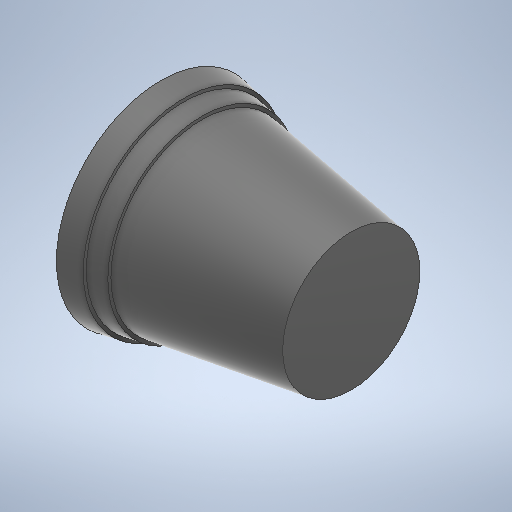
# Autodesk Inventor part: Tanque
Saved by Autodesk Inventor 2025.3 (Build 293356000, 356)
## iProperties
Created: 2025-11-02
Part Number: Tanque
Material: Plástico ABS
Document SubType Name: Modeling
Designer: PAVILION
Density: 1.06 g/cm^3
Appearance: Suave - Blanco
Author: PAVILION
Autodesk Inventor part; units mm, degrees
ref_plane "YZ Plane" through (0, 0, 0) normal (1, 0, 0) x (0, 1, 0)
ref_plane "XZ Plane" through (0, 0, 0) normal (0, 1, 0) x (-1, 0, 0)
ref_plane "XY Plane" through (0, 0, 0) normal (0, 0, 1) x (1, 0, 0)
sketch "Boceto1" plane through (0, 0, 0) normal (0, 1, 0) x (-1, 0, 0)
  line L0 (0, 450) -> (0, -450)
  line L1 (1250, 685) -> (1250, -685)
  line L2 (1250, 685) -> (1100, 658.551)
  line L3 (1100, 658.551) -> (1100, 638.551)
  line L4 (1100, 638.551) -> (980, 617.3917)
  line L5 (980, 617.3917) -> (980, 597.3917)
  line L6 (980, 597.3917) -> (0, 450)
  line L7 (1250, 668.5436) -> (1114.356, 644.6259)
  line L8 (1114.356, 644.6259) -> (1114.356, 624.6259)
  line L9 (1114.356, 624.6259) -> (994.356, 603.4667)
  line L10 (994.356, 603.4667) -> (994.356, 583.4667)
  line L11 (994.356, 583.4667) -> (20, 435)
  line L12 (20, 435) -> (20, 0)
  line L13 (0, 0) -> (20, 0)
  line L14 (1250, 685) -> (1250, 668.5436)
  line L15 (0, 0) -> (1250, 0)
  dimension "d0" = 900
  dimension "d1" = 1370
  dimension "d2" = 1250
  dimension "d3" = 100
  dimension "d4" = 100
  dimension "d5" = 150
  dimension "d6" = 20
  dimension "d7" = 120
  dimension "d8" = 20
  dimension "d9" = 20
  dimension "d11" = 100
  dimension "d12" = 100
  dimension "d13" = 20
  dimension "d14" = 20
  dimension "d15" = 20
  dimension "d18" = 20
  dimension "d19" = 25
  constraints: 32 end point, 4 vertical, 3 parallel, 2 horizontal, 2 midpoint, 1 collinear, 1 horizontal alignment, 1 point on line
  measures "d0" distance of L0.start L0.end
  measures "d1" distance of L1.start L1.end
  measures "d2" distance between parallel lines of L1 L0
  measures "d3" angle of L2 L3
  measures "d4" angle of L4 L5
  measures "d5" horizontal distance of L1.start L2.end
  measures "d6" distance of L2.end L3.end
  measures "d7" horizontal distance of L3.end L4.end
  measures "d8" distance of L4.end L5.end
  measures "d9" distance between parallel lines of L0 L12
  measures "d11" angle of L8 L7
  measures "d12" angle of L9 L10
  measures "d13" distance of L2.end L7.end
  measures "d14" distance of L9.end L4.end
  measures "d15" distance of L5.end L10.end
  measures "d18" distance of L7.end L8.end
  measures "d19" distance of L0.start L11.end
revolve "Revolución1" add sketch "Boceto1" angle 360 about axis through (0, 0, 0) along (-1, 0, 0) contours L6 L5 L4 L3 L2 L1 L7 L8 L9 L10 L11 L12 L13 L0
